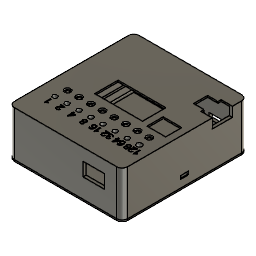
POTYv1.3.2 (Autodesk Fusion 360 design; units mm, degrees)
Autodesk Fusion 360 part; units mm, degrees
sketch "Sketch1" plane through (0, 0, 0) normal (0, 0, 1) x (1, 0, 0)
  circle A0 centre (12.1626, -0.561) radius 2
  line L0 (24.1269, -3.611) -> (30.2269, 2.489) construction
  line L1 (7.7055, -3.611) -> (1.6055, 2.489) construction
  line L2 (16.6197, -3.611) -> (16.6197, 2.489)
  line L3 (-7.3088, 2.489) -> (-7.3088, -3.611)
  line L4 (0.1983, -3.611) -> (-5.9017, 2.489) construction
  line L5 (30.2269, 2.489) -> (30.2269, -3.611)
  line L6 (1.6055, -3.611) -> (7.7055, 2.489) construction
  circle A1 centre (-25.3731, -0.561) radius 2
  line L7 (16.6197, 2.489) -> (22.7197, 2.489)
  line L8 (-14.816, 2.489) -> (-14.816, -3.611)
  line L9 (-5.9017, -3.611) -> (0.1983, 2.489) construction
  line L10 (-7.3088, 2.489) -> (-7.3088, -3.611)
  line L11 (-13.4088, 2.489) -> (-7.3088, 2.489)
  line L12 (-5.9017, -3.611) -> (-5.9017, 2.489)
  line L13 (30.2269, -3.611) -> (24.1269, 2.489) construction
  line L14 (30.2269, -3.611) -> (24.1269, 2.489) construction
  line L15 (-13.4088, -3.611) -> (-13.4088, 2.489)
  line L16 (9.1126, -3.611) -> (15.2126, 2.489) construction
  line L17 (1.6055, -3.611) -> (1.6055, 2.489)
  line L18 (-5.9017, -3.611) -> (0.1983, 2.489) construction
  line L19 (-28.4231, -3.611) -> (-28.4231, 2.489)
  line L20 (-28.4231, -3.611) -> (-22.3231, 2.489) construction
  line L21 (9.1126, -3.611) -> (15.2126, 2.489) construction
  line L22 (-14.816, 2.489) -> (-14.816, -3.611)
  line L23 (-14.816, -3.611) -> (-20.916, 2.489) construction
  line L24 (-7.3088, -3.611) -> (-13.4088, -3.611)
  line L25 (12.1625, -3.561) -> (12.1626, -0.561)
  circle A2 centre (-10.5945, -7.961) radius 1.5
  line L26 (-7.3088, -3.611) -> (-13.4088, -3.611)
  line L27 (-10.3589, -3.561) -> (-10.3588, -0.561)
  line L28 (-2.8518, -3.561) -> (-2.8517, -0.561)
  line L29 (-17.8661, -3.561) -> (-17.866, -0.561)
  line L30 (-22.3231, -3.611) -> (-28.4231, -3.611)
  line L31 (30.2269, -3.611) -> (24.1269, -3.611)
  line L32 (27.1768, -3.561) -> (27.1769, -0.561)
  line L33 (-14.816, -3.611) -> (-20.916, -3.611)
  line L34 (-14.816, -3.611) -> (-20.916, -3.611)
  line L35 (4.6554, -3.561) -> (4.6555, -0.561)
  line L36 (7.7055, -3.611) -> (1.6055, -3.611)
  line L37 (28.4769, -7.961) -> (28.4769, -7.5591)
  line L38 (22.7197, -3.611) -> (16.6197, -3.611)
  line L39 (-17.8661, -3.561) -> (-17.866, -0.561)
  line L40 (-10.3589, -3.561) -> (-10.3588, -0.561)
  circle A3 centre (12.6483, -7.961) radius 1.5
  line L41 (27.1768, -3.561) -> (27.1769, -0.561)
  line L42 (-25.3732, -3.561) -> (-25.3731, -0.561)
  line L43 (-22.3231, -3.611) -> (-28.4231, -3.611)
  circle A4 centre (90.2626, -7.961) radius 1.5
  line L44 (7.7055, -3.611) -> (1.6055, -3.611)
  line L45 (30.2269, -3.611) -> (24.1269, -3.611)
  line L46 (19.6697, -3.561) -> (19.6697, -0.561)
  line L47 (-2.8518, -3.561) -> (-2.8517, -0.561)
  line L48 (22.7197, -3.611) -> (16.6197, -3.611)
  line L49 (-25.3732, -3.561) -> (-25.3731, -0.561)
  circle A5 centre (-18.3088, -7.961) radius 1.5
  circle A6 centre (-2.8803, -7.961) radius 1.5
  line L50 (19.6697, -3.561) -> (19.6697, -0.561)
  circle A7 centre (20.5626, -7.961) radius 1.5
  circle A8 centre (4.834, -7.961) radius 1.5
  line L51 (15.2126, -3.611) -> (9.1126, -3.611)
  line L52 (28.4769, -7.961) -> (28.4769, -6.461)
  line L53 (-5.9017, 2.489) -> (0.1983, 2.489)
  line L54 (-20.916, -3.611) -> (-20.916, 2.489)
  line L55 (-5.9017, 2.489) -> (0.1983, 2.489)
  line L56 (-13.4088, -3.611) -> (-7.3088, 2.489) construction
  line L57 (22.7197, 2.489) -> (22.7197, -3.611)
  line L58 (15.2126, 2.489) -> (15.2126, -3.611)
  line L59 (9.1126, 2.489) -> (15.2126, 2.489)
  circle A9 centre (4.6555, -0.561) radius 2
  line L60 (24.1269, -3.611) -> (24.1269, 2.489)
  line L61 (0.1983, -3.611) -> (-5.9017, 2.489) construction
  circle A10 centre (-10.3588, -0.561) radius 2
  line L62 (22.7197, 2.489) -> (22.7197, -3.611)
  line L63 (0.1983, 2.489) -> (0.1983, -3.611)
  line L64 (15.2126, -3.611) -> (9.1126, 2.489) construction
  circle A11 centre (27.1769, -0.561) radius 2
  line L65 (24.1269, 2.489) -> (30.2269, 2.489)
  line L66 (9.1126, -3.611) -> (9.1126, 2.489)
  line L67 (-28.4231, -3.611) -> (-22.3231, 2.489) construction
  line L68 (-22.3231, 2.489) -> (-22.3231, -3.611)
  line L69 (-22.3231, -3.611) -> (-28.4231, 2.489) construction
  line L70 (-13.4088, 2.489) -> (-7.3088, 2.489)
  line L71 (-28.4231, 2.489) -> (-22.3231, 2.489)
  line L72 (7.7055, 2.489) -> (7.7055, -3.611)
  circle A12 centre (12.1626, -0.561) radius 2
  line L73 (0.1983, 2.489) -> (0.1983, -3.611)
  line L74 (24.1269, -3.611) -> (30.2269, 2.489) construction
  line L75 (16.6197, -3.611) -> (22.7197, 2.489) construction
  line L76 (-7.3088, -3.611) -> (-13.4088, 2.489) construction
  line L77 (-14.816, -3.611) -> (-20.916, 2.489) construction
  line L78 (-28.4231, 2.489) -> (-22.3231, 2.489)
  circle A13 centre (-10.3588, -0.561) radius 2
  line L79 (16.6197, -3.611) -> (16.6197, 2.489)
  line L80 (9.1126, -3.611) -> (9.1126, 2.489)
  line L81 (15.2126, 2.489) -> (15.2126, -3.611)
  line L82 (24.1269, 2.489) -> (30.2269, 2.489)
  line L83 (1.6055, -3.611) -> (1.6055, 2.489)
  line L84 (-22.3231, 2.489) -> (-22.3231, -3.611)
  circle A14 centre (-17.866, -0.561) radius 2
  circle A15 centre (-2.8517, -0.561) radius 2
  line L85 (-20.916, 2.489) -> (-14.816, 2.489)
  line L86 (0.1983, -3.611) -> (-5.9017, -3.611)
  line L87 (9.1126, 2.489) -> (15.2126, 2.489)
  line L88 (16.6197, 2.489) -> (22.7197, 2.489)
  line L89 (0.1983, -3.611) -> (-5.9017, -3.611)
  line L90 (7.7055, -3.611) -> (1.6055, 2.489) construction
  line L91 (1.6055, 2.489) -> (7.7055, 2.489)
  line L92 (1.6055, 2.489) -> (7.7055, 2.489)
  line L93 (12.1625, -3.561) -> (12.1626, -0.561)
  line L94 (-20.916, 2.489) -> (-14.816, 2.489)
  line L95 (15.2126, -3.611) -> (9.1126, -3.611)
  circle A16 centre (-26.1231, -7.961) radius 1.5
  line L96 (4.6554, -3.561) -> (4.6555, -0.561)
  line L97 (-22.3231, -3.611) -> (-28.4231, 2.489) construction
  line L98 (22.7197, -3.611) -> (16.6197, 2.489) construction
  line L99 (-5.9017, -3.611) -> (-5.9017, 2.489)
  circle A17 centre (27.1769, -0.561) radius 2
  circle A18 centre (-25.3731, -0.561) radius 2
  circle A19 centre (-2.8517, -0.561) radius 2
  line L100 (7.7055, 2.489) -> (7.7055, -3.611)
  line L101 (-13.4088, -3.611) -> (-7.3088, 2.489) construction
  line L102 (24.1269, -3.611) -> (24.1269, 2.489)
  line L103 (-20.916, -3.611) -> (-20.916, 2.489)
  circle A20 centre (4.6555, -0.561) radius 2
  line L104 (-20.916, -3.611) -> (-14.816, 2.489) construction
  circle A21 centre (-17.866, -0.561) radius 2
  line L105 (22.7197, -3.611) -> (16.6197, 2.489) construction
  line L106 (-7.3088, -3.611) -> (-13.4088, 2.489) construction
  line L107 (16.6197, -3.611) -> (22.7197, 2.489) construction
  line L108 (-13.4088, -3.611) -> (-13.4088, 2.489)
  line L109 (-20.916, -3.611) -> (-14.816, 2.489) construction
  line L110 (-28.4231, -3.611) -> (-28.4231, 2.489)
  line L111 (15.2126, -3.611) -> (9.1126, 2.489) construction
  line L112 (30.2269, 2.489) -> (30.2269, -3.611)
  circle A22 centre (19.6697, -0.561) radius 2
  line L113 (1.6055, -3.611) -> (7.7055, 2.489) construction
  circle A23 centre (19.6697, -0.561) radius 2
  line L114 (0.1983, 2.489) -> (0.1983, 6.389)
  line L115 (0.1983, 6.389) -> (0.1983, 7.389)
  line L116 (0.1983, 6.389) -> (0.1983, 20.389)
  line L117 (0.1983, 20.389) -> (0.1983, 21.389)
  line L118 (16.6197, 2.489) -> (15.2126, 2.489)
  line L119 (-14.816, 2.489) -> (-14.816, 20.889)
  line L120 (15.9162, 2.489) -> (15.9162, 21.389)
  line L121 (15.9162, 21.389) -> (-14.816, 21.389)
  line L122 (-14.816, 21.389) -> (-14.816, 6.389)
  line L123 (-14.816, 6.389) -> (15.9162, 6.389)
  line L124 (15.9162, 6.389) -> (15.9162, 21.389)
  line L125 (30.2269, 2.489) -> (32.1269, 2.489)
  line L126 (32.1269, 2.489) -> (32.1269, 5.289)
  line L127 (20.1269, 5.289) -> (20.1269, 15.489)
  line L128 (20.1269, 15.489) -> (32.1269, 15.489)
  line L129 (32.1269, 15.489) -> (32.1269, 5.289)
  circle A24 centre (28.0769, -7.861) radius 1.75
  line L130 (20.1269, 5.289) -> (20.1269, 5.089)
  line L131 (20.1269, 5.089) -> (32.1269, 5.089)
  line L132 (15.9162, 21.389) -> (15.9162, 27.689)
  line L133 (20.1269, 15.489) -> (22.5269, 15.489)
  line L134 (22.5269, 15.489) -> (22.5269, 32.689)
  line L135 (22.5269, 32.689) -> (34.5269, 32.689)
  line L136 (34.5269, 32.689) -> (34.5269, 41.689)
  line L137 (34.5269, 41.689) -> (22.5269, 41.689)
  line L138 (22.5269, 41.689) -> (22.5269, 32.689)
  line L139 (30.2269, -3.611) -> (30.2269, -23.311)
  line L140 (34.5269, 32.689) -> (34.5269, -23.311)
  line L141 (34.5269, -23.311) -> (-34.4731, -23.311)
  line L142 (34.5269, 41.689) -> (34.5269, 51.189)
  line L143 (34.5269, 51.189) -> (-34.4731, 51.189)
  line L144 (-34.4731, 51.189) -> (-34.4731, -23.311)
  line L145 (35.5269, 32.689) -> (35.5269, -24.311)
  line L146 (35.5269, -24.311) -> (-35.4731, -24.311)
  line L147 (-35.4731, 52.189) -> (-35.4731, -24.311)
  line L148 (35.5269, 52.189) -> (-35.4731, 52.189)
  line L149 (35.5269, 41.689) -> (35.5269, 52.189)
  line L150 (35.5269, 41.689) -> (34.5269, 41.689)
  line L151 (35.5269, 32.689) -> (34.5269, 32.689)
  line L152 (-28.4231, -3.611) -> (-28.9888, -4.1767)
  line L153 (30.2269, 2.489) -> (30.7926, 3.0546)
  line L154 (-28.9888, -4.1767) -> (30.7926, -4.1767)
  line L155 (30.7926, -4.1767) -> (30.7926, 3.0546)
  line L156 (30.7926, 3.0546) -> (-28.9888, 3.0546)
  line L157 (-28.9888, 3.0546) -> (-28.9888, -4.1767)
  line L158 (-28.4231, -3.611) -> (30.2269, -3.611)
  line L159 (-28.4231, 2.489) -> (30.2269, 2.489)
  circle A25 centre (20.5626, -7.961) radius 1.9
  circle A26 centre (12.6483, -7.961) radius 1.9
  circle A27 centre (4.834, -7.961) radius 1.9
  circle A28 centre (-2.8803, -7.961) radius 1.9
  circle A29 centre (-10.5945, -7.961) radius 1.9
  circle A30 centre (-18.3088, -7.961) radius 1.9
  circle A31 centre (-26.1231, -7.961) radius 1.9
  circle A32 centre (28.0769, -7.861) radius 2.15
  point P0 (27.1769, -0.561)
  point P1 (19.6697, -0.561)
  point P2 (-25.3731, -0.561)
  point P3 (12.1626, -0.561)
  point P4 (4.6555, -0.561)
  point P5 (12.1626, -0.561)
  point P6 (27.1769, -0.561)
  point P7 (-10.3588, -0.561)
  point P8 (4.6555, -0.561)
  point P9 (19.6697, -0.561)
  point P10 (-25.3731, -0.561)
  point P11 (-17.866, -0.561)
  point P12 (-10.3588, -0.561)
  point P13 (-2.8517, -0.561)
  point P14 (-2.8517, -0.561)
  point P15 (-17.866, -0.561)
  dimension "d37" = 52.55
  dimension "d38" = 0
  dimension "d45" = 52.55
  dimension "d46" = 0
  dimension "d48" = 3
  dimension "d49" = 4
  dimension "d50" = 6.1
  dimension "d51" = 6.1
  dimension "d52" = 3
  dimension "d53" = 3
  dimension "d54" = 4
  dimension "d55" = 6.1
  dimension "d56" = 6.1
  dimension "d57" = 3.9
  dimension "d58" = 1
  dimension "d59" = 14
  dimension "d60" = 1
  dimension "d61" = 1.9
  dimension "d63" = 12
  dimension "d64" = 10.2
  dimension "d79" = 0.2
  dimension "d80" = 2.6
  dimension "d81" = 6.3
  dimension "d82" = 2.4
  dimension "d83" = 17.2
  dimension "d84" = 12
  dimension "d85" = 9
  dimension "d86" = 19.7
  dimension "d87" = 69
  dimension "d88" = 9.5
  dimension "d89" = -1
  dimension "d90" = 0.8
  dimension "d91" = 0.8
  dimension "d115" = 3.8
  dimension "d116" = 3.8
  dimension "d117" = 3.8
  dimension "d118" = 3.8
  dimension "d119" = 3.8
  dimension "d120" = 3.8
  dimension "d121" = 3.8
  dimension "d122" = 4.3
  constraint coincident P10 P2
  constraint horizontal L43
  constraint perpendicular L19 L43
  constraint parallel L43 L71
  constraint parallel L19 L68
  constraint coincident P10 L97
  constraint coincident P10 L20
  constraint vertical L52
  constraint horizontal L30
  constraint perpendicular L30 L110
  constraint parallel L30 L78
  constraint parallel L84 L110
  constraint coincident P10 L69
  constraint coincident P10 L67
  constraint coincident L37.end L52
  constraint perpendicular L53 L114
  constraint perpendicular L55 L115
  constraint parallel L115 L116
  constraint parallel L116 L117
  constraint perpendicular L85 L119
  constraint midpoint L118 L120.start
  constraint perpendicular L118 L120
  constraint horizontal L121
  constraint vertical L122
  constraint horizontal L123
  constraint vertical L124
  constraint coincident L119 L122.end
  constraint perpendicular L112 L125
  constraint perpendicular L125 L126
  constraint perpendicular L127 L128
  constraint coincident L126 L131.end
  constraint perpendicular L126 L131
  constraint perpendicular L121 L132
  constraint coincident L128 L133.end
  constraint perpendicular L124 L133
  constraint perpendicular L133 L134
  constraint horizontal L135
  constraint vertical L136
  constraint horizontal L137
  constraint vertical L138
  constraint perpendicular L45 L139
  constraint perpendicular L135 L140
  constraint perpendicular L140 L141
  constraint perpendicular L137 L142
  constraint perpendicular L142 L143
  constraint perpendicular L141 L144
  constraint perpendicular L142 L150
  constraint perpendicular L136 L151
  constraint parallel L20 L152
  constraint parallel L74 L153
  constraint horizontal L154
  constraint vertical L155
  constraint horizontal L156
  constraint vertical L157
  constraint concentric A7 A25
  constraint concentric A3 A26
  constraint concentric A8 A27
  constraint concentric A6 A28
  constraint concentric A2 A29
  constraint concentric A5 A30
  constraint concentric A16 A31
  constraint concentric A24 A32
  measures "d48" distance of L42.start P10
  measures "d49" diameter of A1
  measures "d50" distance of L20.end L19.end
  measures "d51" distance of L19.start L19.end
  measures "d52" diameter of A16
  measures "d53" distance of L42.start P10
  measures "d54" diameter of A18
  measures "d55" distance of L20.end L19.end
  measures "d56" distance of L19.end L19.start
  measures "d57" distance of L9.end L114.end
  measures "d58" distance of L114.end L115.end
  measures "d59" distance of L114.end L116.end
  measures "d60" distance of L116.end L117.end
  measures "d61" distance of L0.end L125.end
  measures "d63" distance of L126.end L127.start
  measures "d64" distance of L127.start L127.end
  measures "d79" distance of L127.start L130.end
  measures "d80" distance of L82 L131
  measures "d81" distance of L120.end L132.end
  measures "d82" distance of L127.end L133.end
  measures "d83" distance of L133.end L134.end
  measures "d84" distance of L134.end L135.end
  measures "d85" distance of L134.end L137.end
  measures "d86" distance of L5.end L139.end
  measures "d87" distance of L140.end L141.end
  measures "d88" distance of L136.end L142.end
  measures "d90" distance of L19.start L152.end
  measures "d91" distance of L0.end L153.end
  measures "d115" diameter of A25
  measures "d116" diameter of A26
  measures "d117" diameter of A27
  measures "d118" diameter of A28
  measures "d119" diameter of A29
  measures "d120" diameter of A30
  measures "d121" diameter of A31
  measures "d122" diameter of A32
extrude "Extrude7" add sketch "Sketch1" along normal blind 1 contours L2 L58 L79 L81 L118 L158 L159 | L2 L7 L38 L48 L57 L62 L79 L88 L158 L159 | L24 L26 L30 L31 L33 L34 L36 L38 L43 L44 L45 L48 L51 L86 L89 L95 L139 L152 L154 L158 | L7 L65 L82 L88 L118 L120 L153 L156 L159 | L57 L60 L62 L102 L158 L159 | L51 L58 L59 L66 L80 L81 L87 L95 L158 L159 | L59 L87 L91 L92 L114 L118 L120 L156 L159 | L5 L31 L45 L60 L65 L82 L102 L112 L158 L159 | L66 L72 L80 L100 L158 L159 | L114 L120 L123 L156 | A32 | L119 L120 L121 L122 L124 L125 L126 L127 L128 L130 L131 L133 L134 L137 L138 L139 L141 L142 L143 L144 L154 L155 L156 L157 | L5 L112 L125 L139 L154 L155 | L17 L36 L44 L72 L83 L91 L92 L100 L158 L159 | L125 L153 L155 | L114 L119 L123 L156 | L11 L53 L55 L70 L114 L119 L156 L159 | L125 L126 L128 L129 L134 L135 L139 L140 L141 L154 L155 | L17 L63 L73 L83 L158 L159 | L12 L53 L55 L63 L73 L86 L89 L99 L158 L159 | L19 L71 L78 L85 L94 L110 L119 L152 L156 L157 L159 | L3 L10 L12 L99 L158 L159 | L8 L15 L22 L108 L158 L159 | L8 L22 L33 L34 L54 L85 L94 L103 L158 L159 | L140 L141 L142 L143 L144 L145 L146 L147 L148 L149 L150 L151 | L19 L30 L43 L68 L71 L78 L84 L110 L158 L159 | L3 L10 L11 L15 L24 L26 L70 L108 L158 L159 | L54 L68 L84 L103 L158 L159 | A25 | A26 | A27 | A28 | A29 | A30 | A31 makes body 1
extrude "Extrude8" add sketch "Sketch1" against normal blind 2 contours L2 L58 L79 L81 L118 L158 L159 | L24 L26 L30 L31 L33 L34 L36 L38 L43 L44 L45 L48 L51 L86 L89 L95 L139 L152 L154 L158 | L7 L65 L82 L88 L118 L120 L153 L156 L159 | L57 L60 L62 L102 L158 L159 | L59 L87 L91 L92 L114 L118 L120 L156 L159 | L66 L72 L80 L100 L158 L159 | L5 L112 L125 L139 L154 L155 | L125 L153 L155 | L11 L53 L55 L70 L114 L119 L156 L159 | L17 L63 L73 L83 L158 L159 | L19 L71 L78 L85 L94 L110 L119 L152 L156 L157 L159 | L3 L10 L12 L99 L158 L159 | L8 L15 L22 L108 L158 L159 | L54 L68 L84 L103 L158 L159 bodies 1
extrude "Extrude9" add sketch "Sketch1" against normal blind 6 contours L140 L141 L142 L143 L144 L145 L146 L147 L148 L149 L150 L151 bodies 1
extrude "Extrude10" add 1 faces at (-9.0617, -4.1767, -0.6667) along direction (0, -1, 0) blind 0.6 on bodies 1 bodies 1
extrude "Extrude11" add 1 faces at (10.8654, 3.0546, -0.6667) along direction (0, 1, 0) blind 0.6 on bodies 1 bodies 1
extrude "Extrude12" add 1 faces at (-28.9888, 0.8442, -0.6667) along direction (-1, 0, 0) blind 2 on bodies 1 bodies 1
extrude "Extrude13" add 1 faces at (30.7926, -1.9663, -0.6667) along direction (1, 0, 0) blind 2 on bodies 1 bodies 1
sketch "Sketch5" plane through (0, 0, 0) normal (0, 0, -1) x (1, 0, 0)
  line L0 (32.7926, -3.6546) -> (-30.9888, -3.6546)
  line L1 (-30.9888, -3.6546) -> (-30.9888, 4.7767)
  line L2 (-30.9888, 4.7767) -> (32.7926, 4.7767)
  line L3 (32.7926, 4.7767) -> (32.7926, -3.6546)
  circle A0 centre (28.0769, 7.861) radius 1.75
  circle A1 centre (12.6483, 7.961) radius 1.5
  line L4 (15.9162, -6.389) -> (15.9162, -21.389)
  line L5 (15.9162, -21.389) -> (-14.816, -21.389)
  line L6 (-14.816, -21.389) -> (-14.816, -6.389)
  line L7 (-14.816, -6.389) -> (15.9162, -6.389)
  line L8 (20.1269, -15.489) -> (20.1269, -5.089)
  line L9 (20.1269, -5.089) -> (32.1269, -5.089)
  line L10 (32.1269, -5.089) -> (32.1269, -15.489)
  line L11 (32.1269, -15.489) -> (20.1269, -15.489)
  circle A2 centre (20.5626, 7.961) radius 1.5
  circle A3 centre (-18.3088, 7.961) radius 1.5
  circle A4 centre (-2.8803, 7.961) radius 1.5
  circle A5 centre (-10.5945, 7.961) radius 1.5
  circle A6 centre (4.834, 7.961) radius 1.5
  circle A7 centre (-26.1231, 7.961) radius 1.5
  line L12 (34.5269, -51.189) -> (34.5269, -41.689)
  line L13 (34.5269, -41.689) -> (22.5269, -41.689)
  line L14 (22.5269, -41.689) -> (22.5269, -32.689)
  line L15 (22.5269, -32.689) -> (34.5269, -32.689)
  line L16 (34.5269, -32.689) -> (34.5269, 23.311)
  line L17 (34.5269, 23.311) -> (-34.4731, 23.311)
  line L18 (-34.4731, 23.311) -> (-34.4731, -51.189)
  line L19 (-34.4731, -51.189) -> (34.5269, -51.189)
  circle A8 centre (-27, -45) radius 3.5
  line L20 (-30, -11) -> (-24, -11)
  line L21 (-24, -11) -> (-24, -13)
  line L22 (-24, -13) -> (-30, -13)
  line L23 (-30, -13) -> (-30, -11)
  dimension "d110" = 7
  constraint horizontal L20
  constraint vertical L21
  constraint horizontal L22
  constraint vertical L23
  measures "d110" diameter of A8
extrude "Extrude15" add sketch "Sketch5" along normal blind 5.9 contours A8 | L20 L21 L22 L23 bodies 1
fillet "Fillet2" radius 1 1 edges at (-30.2631, 46.2657, -5.9) on bodies 1
move_face "MoveFace1" by (0, -2, 0) 2 faces at (11.5269, -23.311, -2) (-11.8065, -24.311, -3.6667) on bodies 1
extrude "Extrude16" add sketch "Sketch1" against normal blind 1.5 contours A32 | A25 | A26 | A27 | A28 | A29 | A30 | A31 bodies 1
fillet "Fillet3" radius 2 1 edges at (-30.2631, 43.7343, 0) on bodies 1
fillet "Fillet4" radius 1.5 4 edges at (-27, 13, 0) (-24, 12, 0) (-27, 11, 0) (-30, 12, 0) on bodies 1
sketch "Sketch6" plane through (0, 0, 1) normal (0, 0, 1) x (-1, 0, 0)
  circle A0 centre (2.8517, 0.561) radius 2
  circle A1 centre (-12.6483, 7.961) radius 1.5
  circle A2 centre (-19.6697, 0.561) radius 2
  circle A3 centre (-20.5626, 7.961) radius 1.5
  circle A4 centre (17.866, 0.561) radius 2
  circle A5 centre (2.8803, 7.961) radius 1.5
  circle A6 centre (-4.834, 7.961) radius 1.5
  circle A7 centre (-12.1626, 0.561) radius 2
  circle A8 centre (-27.1769, 0.561) radius 2
  line L0 (-20.1269, -5.089) -> (-20.1269, -15.489)
  line L1 (-20.1269, -15.489) -> (-32.1269, -15.489)
  line L2 (-32.1269, -15.489) -> (-32.1269, -5.089)
  line L3 (-32.1269, -5.089) -> (-20.1269, -5.089)
  circle A9 centre (10.3588, 0.561) radius 2
  circle A10 centre (25.3731, 0.561) radius 2
  circle A11 centre (26.1231, 7.961) radius 1.5
  circle A12 centre (-4.6555, 0.561) radius 2
  circle A13 centre (10.5945, 7.961) radius 1.5
  circle A14 centre (18.3088, 7.961) radius 1.5
  line L4 (-15.9162, -21.389) -> (-15.9162, -6.389)
  line L5 (-15.9162, -6.389) -> (14.816, -6.389)
  line L6 (14.816, -6.389) -> (14.816, -21.389)
  line L7 (14.816, -21.389) -> (-15.9162, -21.389)
  circle A15 centre (-28.0769, 7.861) radius 1.75
  line L8 (-35.5269, 26.311) -> (-35.5269, -32.689)
  line L9 (-35.5269, -32.689) -> (-22.5269, -32.689)
  line L10 (-22.5269, -32.689) -> (-22.5269, -41.689)
  line L11 (-22.5269, -41.689) -> (-35.5269, -41.689)
  line L12 (-35.5269, -41.689) -> (-35.5269, -52.189)
  line L13 (-35.5269, -52.189) -> (35.4731, -52.189)
  line L14 (35.4731, -52.189) -> (35.4731, 26.311)
  line L15 (35.4731, 26.311) -> (-35.5269, 26.311)
  line L16 (24.7813, 10.7162) -> (28.7813, 10.7162) construction
  line L17 (28.7813, 10.7162) -> (28.7813, 14.7162) construction
  line L18 (28.7813, 14.7162) -> (24.7813, 14.7162) construction
  line L19 (24.7813, 14.7162) -> (24.7813, 10.7162) construction
  line L20 (17.0674, 10.6043) -> (21.0674, 10.6043) construction
  line L21 (21.0674, 10.6043) -> (21.0674, 14.6043) construction
  line L22 (21.0674, 14.6043) -> (17.0674, 14.6043) construction
  line L23 (17.0674, 14.6043) -> (17.0674, 10.6043) construction
  line L24 (9.1044, 10.6878) -> (13.1044, 10.6878) construction
  line L25 (13.1044, 10.6878) -> (13.1044, 14.6878) construction
  line L26 (13.1044, 14.6878) -> (9.1044, 14.6878) construction
  line L27 (9.1044, 14.6878) -> (9.1044, 10.6878) construction
  line L28 (1.54, 10.8691) -> (5.54, 10.8691) construction
  line L29 (5.54, 10.8691) -> (5.54, 14.8691) construction
  line L30 (5.54, 14.8691) -> (1.54, 14.8691) construction
  line L31 (1.54, 14.8691) -> (1.54, 10.8691) construction
  line L32 (-7.2187, 10.7162) -> (-3.2187, 10.7162) construction
  line L33 (-3.2187, 10.7162) -> (-3.2187, 14.7162) construction
  line L34 (-3.2187, 14.7162) -> (-7.2187, 14.7162) construction
  line L35 (-7.2187, 14.7162) -> (-7.2187, 10.7162) construction
  line L36 (-15.1367, 10.6784) -> (-11.1367, 10.6784) construction
  line L37 (-11.1367, 10.6784) -> (-11.1367, 14.6784) construction
  line L38 (-11.1367, 14.6784) -> (-15.1367, 14.6784) construction
  line L39 (-15.1367, 14.6784) -> (-15.1367, 10.6784) construction
  line L40 (-22.6545, 10.6973) -> (-18.6545, 10.6973) construction
  line L41 (-18.6545, 10.6973) -> (-18.6545, 14.6973) construction
  line L42 (-18.6545, 14.6973) -> (-22.6545, 14.6973) construction
  line L43 (-22.6545, 14.6973) -> (-22.6545, 10.6973) construction
  line L44 (-32.4598, 10.7067) -> (-28.4598, 10.7067) construction
  line L45 (-28.4598, 10.7067) -> (-28.4598, 14.7067) construction
  line L46 (-28.4598, 14.7067) -> (-32.4598, 14.7067) construction
  line L47 (-32.4598, 14.7067) -> (-32.4598, 10.7067) construction
  dimension "d129" = 4
  dimension "d130" = 0
  dimension "d131" = 4
  dimension "d133" = 4
  dimension "d134" = 0
  dimension "d135" = 4
  dimension "d137" = 4
  dimension "d138" = 0
  dimension "d139" = 4
  dimension "d140" = 0
  dimension "d141" = 4
  dimension "d143" = 4
  dimension "d144" = 0
  text T0 "1" font "Arial" height 4 align left top in box 4 x 4 at (24.7813, 10.7162) x (1, 0) y (0, 1) spacing 1 kerned
  text T1 "2\n" font "Arial" height 4 align left top in box 4 x 4 at (17.0674, 10.6043) x (1, 0) y (0, 1) spacing 1 kerned
  text T2 "4" font "Arial" height 4 align left top in box 4 x 4 at (9.1044, 10.6878) x (1, 0) y (0, 1) spacing 1 kerned
  text T3 "8\n" font "Arial" height 4 align left top in box 4 x 4 at (1.54, 10.8691) x (1, 0) y (0, 1) spacing 1 kerned
  text T4 "16" font "Arial" height 4 align left top in box 4 x 4 at (-7.2187, 10.7162) x (1, 0) y (0, 1) spacing 1 kerned
  text T5 "32" font "Arial" height 4 align left top in box 4 x 4 at (-15.1367, 10.6784) x (1, 0) y (0, 1) spacing 1 kerned
  text T6 "64\n" font "Arial" height 4 align left top in box 4 x 4 at (-22.6545, 10.6973) x (1, 0) y (0, 1) spacing 1 kerned
  text T7 "128" font "Arial" height 4 align left top in box 4 x 4 at (-32.4598, 10.7067) x (1, 0) y (0, 1) spacing 1 kerned
extrude "Extrude17" cut sketch "Sketch6" against normal blind 0.5 text T7 T6 T5 T4 T3 T2 T1 T0 bodies 1
sketch "Sketch7" plane through (35.5269, 0, 0) normal (1, 0, 0) x (0, 1, 0)
  line L0 (52.189, -6) -> (52.189, 1)
  line L1 (52.189, 1) -> (41.689, 1)
  line L2 (41.689, 1) -> (41.689, -6)
  line L3 (41.689, -6) -> (52.189, -6)
  line L4 (41.689, 1) -> (32.689, 1)
  line L5 (32.689, 1) -> (32.689, -5.2)
  line L6 (32.689, -5.2) -> (41.689, -5.2)
  line L7 (41.689, -5.2) -> (41.689, 1)
  line L8 (41.689, -5.2) -> (42.689, -5.2)
  line L9 (42.689, -5.2) -> (42.689, 1)
  line L10 (42.689, 1) -> (41.689, 1)
  line L11 (41.689, 1) -> (41.689, -5.2)
  line L12 (32.689, -5.2) -> (31.689, -5.2)
  line L13 (31.689, -5.2) -> (31.689, 1)
  line L14 (31.689, 1) -> (32.689, 1)
  line L15 (32.689, 1) -> (32.689, -5.2)
  dimension "d147" = 9
  dimension "d148" = 6.2
  dimension "d149" = 1
  dimension "d150" = 6.2
  dimension "d151" = 1
  constraint horizontal L4
  constraint vertical L5
  constraint horizontal L6
  constraint vertical L7
  constraint coincident L1.end L2.start
  constraint horizontal L8
  constraint vertical L9
  constraint horizontal L10
  constraint vertical L11
  constraint horizontal L12
  constraint vertical L13
  constraint horizontal L14
  constraint vertical L15
  measures "d147" distance of L1.end L4.end
  measures "d148" distance of L1.end L6.end
  measures "d149" distance of L6.end L8.end
  measures "d150" distance of L6.end L1.end
  measures "d151" distance of L5.end L12.end
extrude "Extrude18" cut sketch "Sketch7" against normal blind 6.3 contours L1 L2 L7 L8 L9 L10 L11 | L2 L4 L5 L6 L7 L11 L15 | L5 L12 L13 L14 L15 bodies 1
extrude "Extrude19" add 1 faces at (34.8602, 32.689, -5.7333) along direction (0, 1, 0) blind 11 on bodies 1 bodies 1
extrude "Extrude20" add 1 faces at (35.1935, 25.689, -6) along direction (0, 0, -1) blind 22 on bodies 1 bodies 1
sketch "Sketch8" plane through (0, -26.311, 0) normal (0, -1, 0) x (1, 0, 0)
  line L0 (35.5269, -28) -> (35.5269, 1)
  line L1 (35.5269, 1) -> (-35.4731, 1)
  line L2 (-35.4731, 1) -> (-35.4731, -28)
  line L3 (-35.4731, -28) -> (35.5269, -28)
  line L4 (25, -15) -> (11.5, -15)
  line L5 (11.5, -15) -> (11.5, -6.8)
  line L6 (11.5, -6.8) -> (25, -6.8)
  line L7 (25, -6.8) -> (25, -15)
  dimension "d158" = 13.5
  dimension "d159" = 8.2
  constraint horizontal L4
  constraint vertical L5
  constraint horizontal L6
  constraint vertical L7
  measures "d158" distance of L4.start L4.end
  measures "d159" distance of L4.start L6.end
extrude "Extrude21" cut sketch "Sketch8" against normal blind 2 contours L4 L5 L6 L7 bodies 1
sketch "Sketch9" plane through (0, 52.189, 0) normal (0, 1, 0) x (-1, 0, 0)
  line L0 (35.4731, -28) -> (35.4731, 1)
  line L1 (35.4731, 1) -> (-35.5269, 1)
  line L2 (-35.5269, 1) -> (-35.5269, -28)
  line L3 (-35.5269, -28) -> (35.4731, -28)
  line L4 (-14, -21) -> (-22.9, -21)
  line L5 (-22.9, -21) -> (-22.9, -17.5)
  line L6 (-22.9, -17.5) -> (-14, -17.5)
  line L7 (-14, -17.5) -> (-14, -21)
  circle A0 centre (-9.4363, -19.5341) radius 1.5
  dimension "d162" = 8.9
  dimension "d163" = 3.5
  dimension "d166" = 3
  constraint horizontal L4
  constraint vertical L5
  constraint horizontal L6
  constraint vertical L7
  measures "d162" distance of L4.start L4.end
  measures "d163" distance of L4.start L6.end
  measures "d166" diameter of A0
extrude "Extrude22" cut sketch "Sketch9" against normal blind 4 contours L4 L5 L6 L7 bodies 1
extrude "Extrude23" cut sketch "Sketch9" against normal blind 3 contours A0 bodies 1
move_face "OffsetFaces1" offset 1 3 faces at (-35.4731, -0.1444, -18.3333) (-19.8154, -26.311, -14) (35.5269, -6.9777, -10.7333) on bodies 1
move_face "OffsetFaces2" offset 1 1 faces at (-21.6478, 52.189, -15.364) on bodies 1
fillet "Fillet5" radius 3.5 4 edges at (36.5269, 53.189, -13.5) (36.5269, -27.311, -13.5) (-36.4731, -27.311, -13.5) (-36.4731, 53.189, -13.5) on bodies 1
extrude "Extrude24" cut 1 faces at (35.8602, 31.689, -1.4) along direction (0, -1, 0) blind 1 on bodies 1 bodies 1
extrude "Extrude25" cut 1 faces at (35.8602, 42.689, -1.4) along direction (0, 1, 0) blind 1 on bodies 1 bodies 1
sketch "Sketch10" plane through (0, 0, -28) normal (0, 0, -1) x (1, 0, 0)
  arc A0 (-36.4731, -49.689) -> (-32.9731, -53.189) centre (-32.9731, -49.689) ccw
  line L0 (-32.9731, -53.189) -> (33.0269, -53.189)
  arc A1 (33.0269, -53.189) -> (36.5269, -49.689) centre (33.0269, -49.689) ccw
  line L1 (36.5269, -49.689) -> (36.5269, 23.811)
  arc A2 (36.5269, 23.811) -> (33.0269, 27.311) centre (33.0269, 23.811) ccw
  line L2 (33.0269, 27.311) -> (-32.9731, 27.311)
  arc A3 (-32.9731, 27.311) -> (-36.4731, 23.811) centre (-32.9731, 23.811) ccw
  line L3 (-36.4731, 23.811) -> (-36.4731, -49.689)
  line L4 (34.5269, 25.311) -> (34.5269, -51.189)
  line L5 (34.5269, -51.189) -> (-34.4731, -51.189)
  line L6 (-34.4731, -51.189) -> (-34.4731, 25.311)
  line L7 (-34.4731, 25.311) -> (34.5269, 25.311)
  line L8 (-32.9731, 27.311) -> (33.0269, 27.311)
  line L9 (36.5269, 23.811) -> (36.5269, -49.689)
  line L10 (33.0269, -53.189) -> (-32.9731, -53.189)
  line L11 (-36.4731, -49.689) -> (-36.4731, 23.811)
  arc A4 (33.0269, -53.189) -> (36.5269, -49.689) centre (33.0269, -49.689) ccw
  arc A5 (-36.4731, -49.689) -> (-32.9731, -53.189) centre (-32.9731, -49.689) ccw
  arc A6 (36.5269, 23.811) -> (33.0269, 27.311) centre (33.0269, 23.811) ccw
  arc A7 (-32.9731, 27.311) -> (-36.4731, 23.811) centre (-32.9731, 23.811) ccw
  line L12 (-34.4731, -51.189) -> (34.5269, -51.189)
  line L13 (34.5269, -51.189) -> (34.5269, 25.311)
  line L14 (34.5269, 25.311) -> (-34.4731, 25.311)
  line L15 (-34.4731, 25.311) -> (-34.4731, -51.189)
  dimension "d177" = 3.5
  constraint horizontal L8
  constraint vertical L9
  constraint horizontal L10
  constraint vertical L11
  constraint tangent L9 A4
  constraint tangent L10 A4
  constraint tangent L10 A5
  constraint tangent L11 A5
  constraint equal A4 A5
  constraint tangent L8 A6
  constraint tangent L9 A6
  constraint equal A4 A6
  constraint tangent L8 A7
  constraint tangent L11 A7
  constraint equal A4 A7
  constraint horizontal L12
  constraint vertical L13
  constraint horizontal L14
  constraint vertical L15
  constraint coincident L4.start L7.end
  constraint coincident L5.end L6.start
  measures "d177" radius of A4
extrude "Extrude26" add sketch "Sketch10" along normal blind 1 separate body contours A0 L0 A1 L1 A2 L2 A3 L3 L8 L9 L10 L11 A4 A5 A6 A7 | L4 L5 L6 L7 L12 L13 L14 L15 makes body 2
extrude "Extrude27" add sketch "Sketch10" against normal blind 5 thin wall 1 inside contours L4 L5 L6 L7 L12 L13 L14 L15 bodies 2
sketch "Sketch11" plane through (34.5269, 0, 0) normal (1, 0, 0) x (0, 1, 0)
  line L0 (-25.311, -28) -> (51.189, -28)
  line L1 (51.189, -28) -> (51.189, -23)
  line L2 (51.189, -23) -> (-25.311, -23)
  line L3 (-25.311, -23) -> (-25.311, -28)
  line L4 (51.189, -23) -> (12.939, -23)
  line L5 (12.939, -23) -> (14.939, -23)
  line L6 (14.939, -23) -> (10.939, -23)
  line L7 (10.939, -23) -> (10.939, -28)
  line L8 (10.939, -28) -> (14.939, -28)
  line L9 (14.939, -28) -> (14.939, -23)
  line L10 (10.939, -23) -> (14.939, -23)
  line L11 (14.939, -23) -> (14.939, -21.5)
  line L12 (14.939, -21.5) -> (10.939, -21.5)
  line L13 (10.939, -21.5) -> (10.939, -23)
  line L14 (10.939, -23) -> (8.939, -23)
  line L15 (8.939, -23) -> (8.939, -28)
  line L16 (8.939, -28) -> (10.939, -28)
  line L17 (10.939, -28) -> (10.939, -23)
  line L18 (14.939, -28) -> (16.939, -28)
  line L19 (16.939, -28) -> (16.939, -23)
  line L20 (16.939, -23) -> (14.939, -23)
  line L21 (14.939, -23) -> (14.939, -28)
  dimension "d183" = 2
  dimension "d184" = 4
  dimension "d185" = 1.5
  dimension "d186" = 2
  dimension "d187" = 2
  constraint coincident L1.end L2.start
  constraint midpoint L2 L4.end
  constraint perpendicular L1 L5
  constraint horizontal L6
  constraint vertical L7
  constraint horizontal L8
  constraint vertical L9
  constraint horizontal L10
  constraint vertical L11
  constraint horizontal L12
  constraint vertical L13
  constraint horizontal L14
  constraint vertical L15
  constraint horizontal L16
  constraint vertical L17
  constraint coincident L0 L15.end
  constraint horizontal L18
  constraint vertical L19
  constraint horizontal L20
  constraint vertical L21
  measures "d183" distance of L4.end L5.end
  measures "d184" distance of L5.end L6.end
  measures "d185" distance of L6.end L12.end
  measures "d186" distance of L6.end L14.end
  measures "d187" distance of L8.end L18.end
extrude "Extrude28" cut sketch "Sketch11" against normal blind 81 contours L0 L2 L7 L14 L15 L16 L17 | L0 L2 L4 L9 L18 L19 L20 L21 bodies 2
move_face "OffsetFaces3" offset -0.2 6 faces at (34.5269, 28.3556, -26.3333) (34.5269, -13.8944, -24.6667) (-11.4731, -25.311, -26.3333) (-34.4731, -2.4777, -24.6667) (-34.4731, 28.3556, -24.6667) (11.5269, 51.189, -26.3333) on bodies 2
move_face "OffsetFaces4" offset 0.5 6 faces at (33.5269, -13.2277, -26.3333) (-11.1398, -24.311, -26.3333) (-33.4731, -2.1444, -24.6667) (-33.4731, 39.1056, -26.3333) (11.1935, 50.189, -26.3333) (33.5269, 28.0223, -26.3333) on bodies 2
extrude "Extrude29" add sketch "Sketch11" against normal blind 1 contours L2 L4 L5 L6 L10 L11 L12 L13 bodies 2
extrude "Extrude30" add sketch "Sketch11" along normal blind 2 contours L2 L4 L5 L6 L10 L11 L12 L13 bodies 2
chamfer "Chamfer2" distance 1 angle 65 1 edges at (36.5269, 12.939, -21.5) measured on face at (36.5269, 12.2723, -22) on bodies 2
sketch "Sketch12" plane through (-34.4731, 0, 0) normal (-1, 0, 0) x (0, -1, 0)
  line L0 (-10.939, -28) -> (-10.939, -23)
  line L1 (-10.939, -23) -> (-14.939, -23)
  line L2 (-14.939, -23) -> (-14.939, -28)
  line L3 (-14.939, -28) -> (-10.939, -28)
  line L4 (-10.939, -23) -> (-15, -23)
  line L5 (-15, -23) -> (-15, -21.5)
  line L6 (-15, -21.5) -> (-10.939, -21.5)
  line L7 (-10.939, -21.5) -> (-10.939, -23)
  constraint horizontal L4
  constraint vertical L5
  constraint horizontal L6
  constraint vertical L7
  constraint coincident L0.end L1.start
extrude "Extrude31" add sketch "Sketch12" against normal blind 1 contours L1 L4 L5 L6 L7 bodies 2
extrude "Extrude32" add sketch "Sketch12" along normal blind 2 contours L1 L4 L5 L6 L7 bodies 2
chamfer "Chamfer3" distance 1 angle 65 1 edges at (-36.4731, 12.9695, -21.5) measured on face at (-36.4731, 13.626, -22) on bodies 2
fillet "Fillet6" radius 3 1 edges at (33.5269, 12.939, -28) on bodies 2
fillet "Fillet7" radius 2 1 edges at (-33.4731, 12.939, -28) on bodies 2
fillet "Fillet8" radius 1 5 edges at (-32.9731, 33.314, -28) (0.0269, 49.689, -28) (33.0269, 33.314, -28) (33.0269, -7.436, -28) (0.0269, -23.811, -28) on bodies 2
sketch "Sketch13" plane through (36.5269, 0, 0) normal (1, 0, 0) x (0, 1, 0)
  line L0 (43.689, 1) -> (43.689, -5.2)
  line L1 (43.689, -5.2) -> (30.689, -5.2)
  line L2 (30.689, -5.2) -> (30.689, 1)
  line L3 (30.689, 1) -> (-23.811, 1)
  line L4 (-23.811, 1) -> (-23.811, -28)
  line L5 (-23.811, -28) -> (49.689, -28)
  line L6 (49.689, -28) -> (49.689, 1)
  line L7 (49.689, 1) -> (43.689, 1)
  line L8 (10.3, -21) -> (15.6, -21)
  line L9 (15.6, -21) -> (15.6, -23.1)
  line L10 (15.6, -23.1) -> (10.3, -23.1)
  line L11 (10.3, -23.1) -> (10.3, -21)
  constraint horizontal L8
  constraint vertical L9
  constraint horizontal L10
  constraint vertical L11
extrude "Extrude33" cut sketch "Sketch13" against normal blind 85 contours L8 L9 L10 L11 bodies 1
fillet "Fillet9" radius 1 1 edges at (-34.4731, 12.939, -23) on bodies 2
fillet "Fillet10" radius 1 1 edges at (34.5269, 12.939, -23) on bodies 2
extrude "Extrude34" cut 1 faces at (20.5, -26.6444, -15) along direction (0, 0, -1) blind 0.5 on bodies 1 bodies 1
extrude "Extrude35" cut 1 faces at (11.5, -26.6444, -9.7) along direction (-1, 0, 0) blind 0.2 on bodies 1 bodies 1
equation "d130 = '1'"
equation "d132 = '2 '"
equation "d134 = '4'"
equation "d136 = '8 '"
equation "d138 = '16'"
equation "d140 = '32'"
equation "d142 = '64 '"
equation "d144 = '128'"
